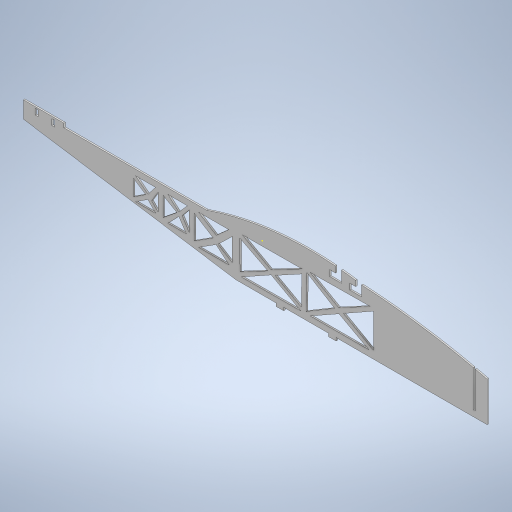
# Autodesk Inventor part: final side pannel
Saved by Autodesk Inventor 2024 (Build 280153000, 153)
## iProperties
Created: 2023-07-19
Part Number: final side pannel
Material: Generic
Document SubType Name: Modeling
Designer: USER
Density: 1 g/cm^3
Appearance: Default
Author: USER
Autodesk Inventor part; units mm, degrees
ref_plane "YZ Plane" through (0, 0, 0) normal (1, 0, 0) x (0, 1, 0)
ref_plane "XZ Plane" through (0, 0, 0) normal (0, 1, 0) x (-1, 0, 0)
ref_plane "XY Plane" through (0, 0, 0) normal (0, 0, 1) x (1, 0, 0)
sketch "Sketch1" plane through (0, 0, 0) normal (0, 0, 1) x (1, 0, 0)
  line L0 (124.0574, 14.5348) -> (114.0574, 14.5348)
  line L1 (114.0574, 14.5348) -> (114.0574, 4.5346)
  line L2 (114.0574, 4.5346) -> (134.0574, 4.5346)
  line L3 (134.0574, 4.5346) -> (134.0574, 23.779)
  arc A0 (158.1943, 20.7355) -> (134.0574, 23.779) centre (79.3774, -507.1118) ccw
  line L4 (158.1943, 20.7355) -> (158.14, 20.7355)
  line L5 (158.14, 20.7355) -> (158.14, 11.7119)
  line L6 (158.14, 11.7119) -> (148.14, 11.7119)
  line L7 (148.14, 11.7119) -> (148.14, 1.7121)
  line L8 (148.14, 1.7121) -> (168.14, 1.7121)
  line L9 (168.14, 1.7121) -> (168.14, 19.1544)
  arc A1 (358.0994, -7.386) -> (168.14, 19.1544) centre (103.4188, -1137.151) ccw
  line L10 (358.0994, -7.386) -> (358.0994, -69.6166)
  line L11 (358.0994, -69.6166) -> (361.0994, -69.6166)
  line L12 (361.0994, -69.6166) -> (361.0994, -8.0665)
  arc A2 (381.0616, -12.8087) -> (361.0994, -8.0665) centre (103.4188, -1137.151) ccw
  line L13 (381.0616, -12.8087) -> (381.1813, -79.5753)
  line L14 (381.1813, -79.5753) -> (281.1815, -79.7546)
  line L15 (281.1815, -79.7546) -> (125.0613, -79.7546)
  line L16 (125.0613, -79.7546) -> (125.0613, -84.8346)
  line L17 (125.0613, -84.8346) -> (112.3613, -84.8346)
  line L18 (112.3613, -84.8346) -> (112.3613, -79.7546)
  line L19 (112.3613, -79.7546) -> (36.1613, -79.7546)
  line L20 (36.1613, -79.7546) -> (36.1613, -84.8346)
  line L21 (36.1613, -84.8346) -> (23.4613, -84.8346)
  line L22 (23.4613, -84.8346) -> (23.4613, -79.7546)
  line L23 (23.4613, -79.7546) -> (-44.8841, -79.7546)
  line L24 (-44.8841, -79.7546) -> (-405.1838, -24.0571)
  line L25 (-405.1838, -24.0571) -> (-405.1838, 4.3589)
  line L26 (-405.1838, 4.3589) -> (-336.4585, 4.3589)
  line L27 (-336.4585, 4.3589) -> (-336.4585, -2.4149)
  line L28 (-336.4585, -2.4149) -> (-94.1621, -2.4149)
  arc A3 (124.0574, 24.7139) -> (-94.1621, -2.4149) centre (79.3774, -507.1118) ccw
  line L29 (124.0574, 24.7139) -> (124.0574, 14.5348)
  line L30 (-197.6668, -31.1888) -> (-218.4818, -17.4299)
  line L31 (-218.4818, -17.4299) -> (-218.4818, -44.8835)
  line L32 (-218.4818, -44.8835) -> (-197.6668, -31.1888)
  line L33 (-215.0181, -12.1898) -> (-193.8383, -28.6699)
  line L34 (-193.8383, -28.6699) -> (-181.015, -12.1898)
  line L35 (-181.015, -12.1898) -> (-215.0181, -12.1898)
  line L36 (-187.5566, -35.167) -> (-176.8518, -46.2388)
  line L37 (-176.8518, -46.2388) -> (-176.8518, -17.4941)
  line L38 (-176.8518, -17.4941) -> (-187.5566, -35.167)
  line L39 (-214.992, -50.1878) -> (-180.9362, -50.1878)
  line L40 (-180.9362, -50.1878) -> (-194.177, -36.4931)
  line L41 (-194.177, -36.4931) -> (-214.992, -50.1878)
  line L42 (-168.3123, -50.1878) -> (-144.7378, -31.1888)
  line L43 (-144.7378, -31.1888) -> (-168.3123, -17.4941)
  line L44 (-168.3123, -17.4941) -> (-168.3123, -50.1878)
  line L45 (-160.0494, -12.1898) -> (-141.6124, -28.6699)
  line L46 (-141.6124, -28.6699) -> (-126.8814, -12.1898)
  line L47 (-126.8814, -12.1898) -> (-160.0494, -12.1898)
  line L48 (-160.0494, -54.317) -> (-128.9473, -54.317)
  line L49 (-128.9473, -54.317) -> (-141.6124, -35.067)
  line L50 (-141.6124, -35.067) -> (-160.0494, -54.317)
  line L51 (-123.9433, -50.1878) -> (-123.9433, -16.6188)
  line L52 (-123.9433, -50.1878) -> (-123.9433, -16.6188)
  line L53 (-123.9433, -16.6188) -> (-135.7178, -31.1888)
  line L54 (-135.7178, -31.1888) -> (-123.9433, -50.1878)
  line L55 (-83.2414, -37.5733) -> (-115.541, -17.4299)
  line L56 (-115.541, -17.4299) -> (-115.541, -58.2492)
  line L57 (-115.541, -58.2492) -> (-83.2414, -37.5733)
  line L58 (-108.0357, -12.1898) -> (-77.8954, -30.9866)
  line L59 (-77.8954, -30.9866) -> (-56.7692, -12.1898)
  line L60 (-56.7692, -12.1898) -> (-108.0357, -12.1898)
  line L61 (-75.0867, -42.6589) -> (-50.9418, -57.7167)
  line L62 (-50.9418, -57.7167) -> (-50.9418, -19.3143)
  line L63 (-50.9418, -19.3143) -> (-75.0867, -42.6589)
  line L64 (-108.0357, -63.7506) -> (-56.4101, -63.7506)
  line L65 (-56.4101, -63.7506) -> (-78.5619, -44.8835)
  line L66 (-78.5619, -44.8835) -> (-108.0357, -63.7506)
  line L67 (-37.8304, -64.8295) -> (9.439, -39.6735)
  line L68 (9.439, -39.6735) -> (-38.0706, -15.2272)
  line L69 (-38.0706, -15.2272) -> (-37.8304, -64.8295)
  line L70 (67.3756, -7.7965) -> (-33.8897, -8.287)
  line L71 (-33.8897, -8.287) -> (14.817, -35.2701)
  line L72 (14.817, -35.2701) -> (67.3756, -7.7965)
  line L73 (67.0354, -15.3008) -> (21.7673, -40.0406)
  line L74 (21.7673, -40.0406) -> (66.1486, -64.432)
  line L75 (66.1486, -64.432) -> (67.0354, -15.3008)
  line L76 (14.9622, -42.7333) -> (-35.4332, -70.9517)
  line L77 (-35.4332, -70.9517) -> (65.0204, -70.4651)
  line L78 (65.0204, -70.4651) -> (14.9622, -42.7333)
  line L79 (122.6917, -37.9612) -> (75.5356, -9.1638)
  line L80 (75.5356, -9.1638) -> (74.3604, -66.7586)
  line L81 (74.3604, -66.7586) -> (122.6917, -37.9612)
  line L82 (182.9351, -5.0105) -> (81.2829, -6.0788)
  line L83 (129.895, -33.6692) -> (182.9351, -5.0105)
  line L84 (182.9351, -5.0105) -> (81.2829, -6.0788)
  line L85 (81.2829, -6.0788) -> (129.895, -33.6692)
  line L86 (188.6122, -66.7586) -> (188.6122, -9.1638)
  line L87 (188.6122, -9.1638) -> (137.6759, -37.9612)
  line L88 (137.6759, -37.9612) -> (188.6122, -66.7586)
  line L89 (180.7186, -69.8436) -> (129.895, -42.3602)
  line L90 (129.895, -42.3602) -> (81.2829, -69.8436)
  line L91 (81.2829, -69.8436) -> (180.7186, -69.8436)
  line L92 (-385.3173, 2.1638) -> (-385.3173, -7.8362)
  line L93 (-385.3173, -7.8362) -> (-380.3173, -7.8362)
  line L94 (-380.3173, -7.8362) -> (-380.3173, 2.1638)
  line L95 (-380.3173, 2.1638) -> (-385.3173, 2.1638)
  line L96 (-356.86, -9.2705) -> (-351.86, -9.2705)
  line L97 (-351.86, -9.2705) -> (-351.86, 0.7295)
  line L98 (-351.86, 0.7295) -> (-356.86, 0.7295)
  line L99 (-356.86, 0.7295) -> (-356.86, -9.2705)
  constraints: 200 end point, 8 centre point, 8 point on circle
extrude "Extrusion1" add sketch "Sketch1" along normal blind 2.5
sketch "Sketch2" plane through (0, 0, 2.5) normal (0, 0, 1) x (1, 0, 0)
  point P0 (0, 0)
body "Solid1"
